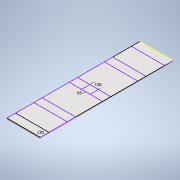
# Autodesk Inventor part: Marcoesumadre
Saved by Autodesk Inventor 2021.2 (Build 252289000, 289)
## iProperties
Created: 2021-04-11
Part Number: Marcoesumadre
Material: Genérico
Document SubType Name: Modeling
Designer: equip
Density: 1 g/cm^3
Appearance: Valor por defecto
Author: equip
Autodesk Inventor part; units mm, degrees
ref_plane "YZ Plane" through (0, 0, 0) normal (1, 0, 0) x (0, 1, 0)
ref_plane "XZ Plane" through (0, 0, 0) normal (0, 1, 0) x (-1, 0, 0)
ref_plane "XY Plane" through (0, 0, 0) normal (0, 0, 1) x (1, 0, 0)
sketch "Boceto1" plane through (0, 0, 0) normal (0, 1, 0) x (-1, 0, 0)
  line L0 (250.06, 997.344) -> (-249.94, 997.344)
  line L1 (-249.94, 997.344) -> (-249.94, -1002.656)
  line L2 (-249.94, -1002.656) -> (250.06, -1002.656)
  line L3 (250.06, -1002.656) -> (250.06, 997.344)
  point P0 (0, 0)
  point P1 (-115.972, 0)
  point P2 (-115.972, 0)
  point P3 (250.06, -1002.656)
  dimension "d0" = 2000
  dimension "d1" = 500
  constraints: 8 end point, 2 parallel, 1 coincident, 1 horizontal, 1 perpendicular
  measures "d0" distance of L3.start L0.start
  measures "d1" distance of L0.end L0.start
extrude "Extrusión1" add sketch "Boceto1" along normal blind 20
sketch "Boceto2" plane through (0, 20, 0) normal (0, 1, 0) x (1, 0, 0)
  line L0 (-250.06, 1002.656) -> (-250.06, -997.344) projected
  line L1 (249.94, 1002.656) -> (-250.06, 1002.656) projected
  line L2 (-250.06, 62.656) -> (-250.06, 467.656)
  line L3 (249.94, -997.344) -> (249.94, 1002.656) projected
  line L4 (-250.06, -997.344) -> (-250.06, -592.344)
  line L5 (-250.06, -592.344) -> (249.94, -592.344)
  line L6 (-250.06, -592.344) -> (-250.06, -467.344)
  line L7 (-250.06, -467.344) -> (249.94, -467.344)
  line L8 (-250.06, -467.344) -> (-250.06, -62.344)
  line L9 (-250.06, -62.344) -> (249.94, -62.344)
  line L10 (-250.06, -62.344) -> (-250.06, 62.656)
  line L11 (-250.06, 62.656) -> (249.94, 62.656)
  line L12 (-250.06, 62.656) -> (-250.06, 467.656)
  line L13 (-250.06, 467.656) -> (249.94, 467.656)
  line L14 (249.94, 1002.656) -> (249.94, -62.344)
  line L15 (249.94, -467.344) -> (249.94, -997.344)
  line L16 (-250.06, 467.656) -> (-250.06, 592.656)
  line L17 (-250.06, 592.656) -> (249.94, 592.656)
  line L18 (-250.06, 592.656) -> (-250.06, 1002.656)
  line L19 (249.94, 1002.656) -> (249.94, -867.344)
  line L20 (-250.06, -997.344) -> (249.94, -997.344) projected
  line L21 (-250.06, -997.344) -> (249.94, -997.344)
  line L22 (-0.06, -62.344) -> (-65.06, -62.344)
  line L23 (-65.06, -62.344) -> (-65.06, 62.656)
  line L24 (-65.06, 62.656) -> (64.94, 62.656)
  line L25 (64.94, 62.656) -> (64.94, -62.344)
  line L26 (249.94, -997.344) -> (249.94, -867.344)
  line L27 (249.94, -867.344) -> (-250.06, -867.344)
  line L28 (249.94, 1002.656) -> (249.94, 872.656)
  line L29 (249.94, 872.656) -> (-250.06, 872.656)
  point P0 (0, 0)
  dimension "d10" = 65
  dimension "d11" = 130
  dimension "d12" = 130
  constraints: 52 end point, 12 perpendicular, 12 point on line, 1 collinear, 1 midpoint, 1 parallel, 1 vertical
  measures "d10" distance of L22.start L22.end
  measures "d11" distance of L23.end L24.end
  measures "d12" distance of L19.end L3.start
